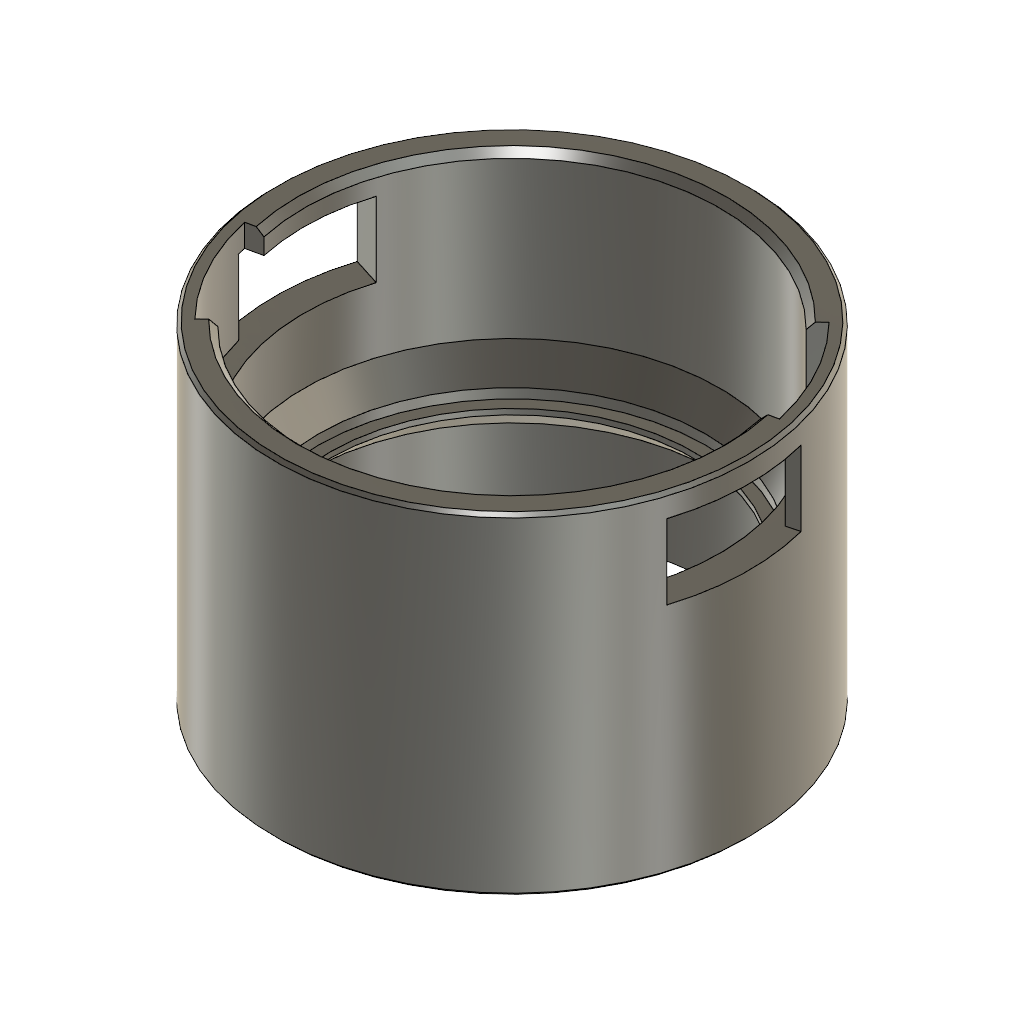
Part3_bayonet_flange (Autodesk Fusion 360 design; units mm, degrees)
part number: 2026-09-28-20-29-22-459
Autodesk Fusion 360 part; units mm, degrees
sketch "Section" plane through (0, 0, 0) normal (0, 1, 0) x (1, 0, 0)
  line L0 (31.65, 0) -> (36, 0)
  line L1 (36, 0) -> (36.5, -0.5)
  line L2 (36.5, -0.5) -> (36.5, -50.5)
  line L3 (36.5, -50.5) -> (36, -51)
  line L4 (36, -51) -> (33, -51)
  line L5 (33, -51) -> (32, -50)
  line L6 (32, -50) -> (32, -26)
  line L7 (32, -26) -> (29.8, -21)
  line L8 (29.8, -21) -> (29.8, -19.5)
  line L9 (29.8, -19.5) -> (28, -19.5)
  line L10 (28, -19.5) -> (28, -18.65)
  line L11 (28, -18.65) -> (31.65, -15)
  line L12 (31.65, -15) -> (31.65, 0)
revolve "Revolve1" add sketch "Section" angle 360 about axis through (0, 0, 1.75) along (0, 0, 1)
ref_plane "WorkPlane1" through (0, 0, 36) normal (0, 0, 1) x (1, 0, 0)
sketch "Windows" plane through (0, 0, 36) normal (0, 0, 1) x (1, 0, 0)
  arc A0 (28.6115, -9.0212) -> (29.0444, 7.5114) centre (0, 0) ccw
  arc A1 (36.7181, -11.5772) -> (37.2737, 9.6396) centre (0, 0) ccw
  line L0 (28.6115, -9.0212) -> (36.7181, -11.5772)
  line L1 (29.0444, 7.5114) -> (37.2737, 9.6396)
  arc A2 (-28.6115, 9.0212) -> (-29.0444, -7.5114) centre (0, 0) ccw
  arc A3 (-36.7181, 11.5772) -> (-37.2737, -9.6396) centre (0, 0) ccw
  line L2 (-28.6115, 9.0212) -> (-36.7181, 11.5772)
  line L3 (-29.0444, -7.5114) -> (-37.2737, -9.6396)
extrude "Windows (1)" cut sketch "Windows" along normal blind 11.5
ref_plane "WorkPlane2" through (0, 0, 36) normal (0, 0, 1) x (1, 0, 0)
sketch "Entry_grooves" plane through (0, 0, 36) normal (0, 0, 1) x (1, 0, 0)
  arc A0 (29.2889, 6.4932) -> (21.3975, 21.0273) centre (0, 0) ccw
  arc A1 (33.6822, 7.4672) -> (24.6071, 24.1814) centre (0, 0) ccw
  line L0 (29.2889, 6.4932) -> (33.6822, 7.4672)
  line L1 (21.3975, 21.0273) -> (24.6071, 24.1814)
  arc A2 (-29.2889, -6.4932) -> (-21.3975, -21.0273) centre (0, 0) ccw
  arc A3 (-33.6822, -7.4672) -> (-24.6071, -24.1814) centre (0, 0) ccw
  line L2 (-29.2889, -6.4932) -> (-33.6822, -7.4672)
  line L3 (-21.3975, -21.0273) -> (-24.6071, -24.1814)
extrude "Entry_grooves (1)" cut sketch "Entry_grooves" along normal blind 16
named bodies: "Part3_bayonet_flange"
